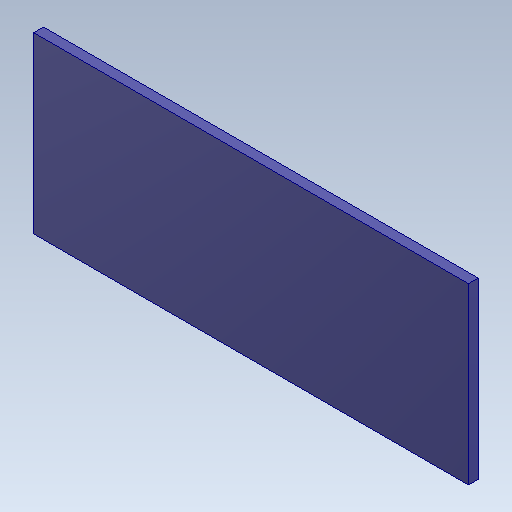
# Autodesk Inventor part: ARDUINO_NANO1_ARDUINO_NANO
Saved by Autodesk Inventor 2020 (Build 240168000, 168)
## iProperties
Created: 2019-07-14
Part Number: ARDUINO_NANO1_ARDUINO_NANO
Material: Generic
Document SubType Name: Modeling
Designer: psrob
Density: 1 g/cm^3
Appearance: ARDUINO_NANO, ARDUINO_NANO1_ARDUINO_NANO
Author: psrob
Autodesk Inventor part; units mm, degrees
ref_plane "YZ Plane" through (0, 0, 0) normal (1, 0, 0) x (0, 1, 0)
ref_plane "XZ Plane" through (0, 0, 0) normal (0, 1, 0) x (-1, 0, 0)
ref_plane "XY Plane" through (0, 0, 0) normal (0, 0, 1) x (1, 0, 0)
sketch "ARDUINO_NANO, ARDUINO_NANO1_ARDUINO_NANO_1" plane through (0, 0, 0) normal (0, 0, 1) x (1, 0, 0)
  line L0 (-25.4, 8.9535) -> (19.1135, 8.9535)
  line L1 (19.1135, 8.9535) -> (19.1135, -8.89)
  line L2 (19.1135, -8.89) -> (-25.4, -8.89)
  line L3 (-25.4, -8.89) -> (-25.4, 8.9535)
  constraints: 8 end point
extrude "Extrusion1" add sketch "ARDUINO_NANO, ARDUINO_NANO1_ARDUINO_NANO_1" along normal blind 1
body "Solid1"
